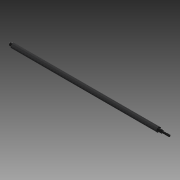
# Autodesk Inventor part: fc18-059
Saved by Autodesk Inventor 2018 (Build 220112000, 112)
## iProperties
Category: Miscellaneous
Company: Autodesk Inc.
Created: 2017-11-24
Part Number: fc18-059
Catalog Web Link: https://us.misumi-ec.com/vona2/detail/110302641830/?OptionSpec=FE%3A%3A0%09FW%3A%3A7%09FY%3A%3A1&CategorySpec=00000029094%3A%3A420&PNSearch=MTSBRK12-420-F7-R8-T9-Q8-S20-E5-FE0-FW7-FY1&SeriesSpec=F%3A%3A7%09R%3A%3A8%09T%3A%3A9%09Q%3A%3A8%09S%3A%3A20%09E%3A%3A5&HissuCode=MTSBRK12-%5B80-1000%2F1%5D-F%5B2-45%2F1%5D-R7%2C8%2C9-T%5B2-45%2F1%5D-Q7%2C8%2C9-S%5B2-40%2F1%5D-E%5B4-8%2F1%5D&KWSearch=MTSBRK12-420-F7-R8-T9-Q8-S20-E5-FE0-FW7-FY1&Keyword=MTSBRK12-420-F7-R8-T9-Q8-S20-E5-FE0-FW7-FY1&searchFlow=results2products&Keyword=MTSBRK12-420-F7-R8-T9-Q8-S20-E5-FE0-FW7-FY1
Description: MTSRK, MTSBRK, RMTSRK, MTSLK, MTSBLK, RMTSLK, MTSWKA, MTSBWKA, RMTSWKA, MTSWKB, MTSBWKB, RMTSWKB-Lead Screws One End Stepped / One End Double Stepped Right-Hand Screw / Left-Hand Screw / Right and Left-Hand Screw 1045 Carbon Steel
Vendor: AndyMark Inc.
Document SubType Name: Modeling
Designer: Autodesk Inc.
Manufacturer: MISUMI
Mass: 350.139 g
Surface Area: 153.947 cm^2
Volume: 44.6037 cm^3
Density: 7.85 g/cm^3
Material: Steel, Carbon
Appearance: Smooth - Black
Title: MTSBRK12-420-F7-R8-T9-Q8-S20-E5-FE0-FW7-FY1
Author: Autodesk Inc.
Comments: Lead Screws One End Stepped / One End Double Stepped Right-Hand Screw / Left-Hand Screw / Right and Left-Hand Screw 1045 Carbon Steel
Keywords: FIRST Choice
Autodesk Inventor part; units mm, degrees
ref_plane "YZ Plane" through (0, 0, 0) normal (1, 0, 0) x (0, 1, 0)
ref_plane "XZ Plane" through (0, 0, 0) normal (0, 1, 0) x (-1, 0, 0)
ref_plane "XY Plane" through (0, 0, 0) normal (0, 0, 1) x (1, 0, 0)
sketch "Sketch_16" plane through (0, 0, 0) normal (0, 0, 1) x (1, 0, 0)
  line L0 (391, 0) -> (7, 0)
  line L1 (7, 0) -> (7, 6)
  line L2 (7, 6) -> (391, 6)
  line L3 (391, 6) -> (391, 0)
  line L4 (391, 0) -> (7, 0)
  constraints: 10 end point
revolve "Revolution1" add sketch "Sketch_16" angle 360 about axis through (391, 0, 0) along (1, 0, 0)
thread "Thread1" size "TR12x2" class "7e" standard "ISO Metric Trapezoidal Threads" full length
sketch "Sketch_23" plane through (0, 0, 0) normal (0, 0, 1) x (1, 0, 0)
  line L0 (7, 0) -> (0, 0)
  line L1 (0, 0) -> (0, 3.5)
  line L2 (0, 3.5) -> (0.5, 4)
  line L3 (0.5, 4) -> (6.7, 4)
  arc A0 (6.7, 4) -> (7, 4.3) centre (6.7, 4.3) ccw
  line L4 (7, 4.3) -> (7, 0)
  line L5 (7, 0) -> (0, 0)
  constraints: 12 end point, 2 point on circle, 1 centre point
revolve "Revolution2" add sketch "Sketch_23" angle 360 about axis through (7, 0, 0) along (1, 0, 0)
sketch "Sketch_4" plane through (0, 0, 0) normal (0, 0, 1) x (1, 0, 0)
  line L0 (420, 0) -> (391, 0)
  line L1 (391, 0) -> (391, 4.3)
  arc A0 (391, 4.3) -> (391.3, 4) centre (391.3, 4.3) ccw
  line L2 (391.3, 4) -> (400, 4)
  line L3 (400, 4) -> (400, 2.8)
  arc A1 (400, 2.8) -> (400.3, 2.5) centre (400.3, 2.8) ccw
  line L4 (400.3, 2.5) -> (419.5, 2.5)
  line L5 (419.5, 2.5) -> (420, 2)
  line L6 (420, 2) -> (420, 0)
  line L7 (420, 0) -> (391, 0)
  constraints: 16 end point, 4 point on circle, 2 centre point
revolve "Revolution3" add sketch "Sketch_4" angle 360 about axis through (420, 0, 0) along (1, 0, 0)
sketch "Sketch_8" plane through (420, 0, 0) normal (1, 0, 0) x (0, 0, -1)
  line L0 (-2.5, -6) -> (-1.5, -6)
  line L1 (-1.5, -6) -> (-1.5, 6)
  line L2 (-1.5, 6) -> (-2.5, 6)
  line L3 (-2.5, 6) -> (-2.5, -6)
  constraints: 8 end point
extrude "Extrusion1" cut sketch "Sketch_8" against normal blind 7
body "Solid1"
